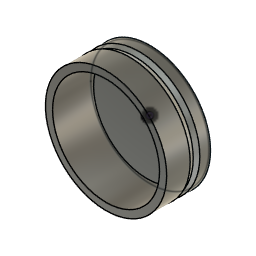
LW_AS_37_0150 (Autodesk Fusion 360 design; units mm, degrees)
Autodesk Fusion 360 part; units mm, degrees
sketch "Sketch1" plane through (0, 0, 0) normal (0, 0, 1) x (1, 0, 0)
  line L0 (0, 0) -> (17, 0)
  line L1 (17, 0) -> (17, -3)
  line L2 (17, -3) -> (17, -5.7)
  line L3 (17, -5.7) -> (17, -12.3)
  line L4 (17, -12.3) -> (15, -12.3)
  line L5 (15, -12.3) -> (15, -0.8)
  line L6 (17, -3) -> (17, -4.35) construction
  line L7 (17, -4.35) -> (16.5, -4.35) construction
  line L8 (17, -3) -> (16.5, -4.35)
  line L9 (16.5, -4.35) -> (17, -5.7)
  line L10 (0, 0) -> (0, -0.8)
  line L11 (0, -0.8) -> (15, -0.8)
  dimension "d1" = 17
  dimension "d2" = 3
  dimension "d4" = 2.7
  dimension "d5" = 6.6
  dimension "d6" = 2
  dimension "d8" = 1.35
  dimension "d9" = 0.5
  dimension "d10" = 15
  dimension "d12" = 17
  dimension "d19" = 0.8
  constraint coincident L0.start L10.start
  constraint horizontal L0
  constraint perpendicular L0 L1
  constraint parallel L1 L2
  constraint parallel L2 L3
  constraint perpendicular L3 L4
  constraint perpendicular L0 L5
  constraint coincident L2 L6.end
  constraint perpendicular L2 L7
  constraint perpendicular L0 L10
  constraint perpendicular L5 L11
  measures "d1" distance of L0.start L0.end
  measures "d2" distance of L0.end L1.end
  measures "d4" distance of L1.end L2.end
  measures "d5" distance of L2.end L3.end
  measures "d6" distance of L3.end L4.end
  measures "d8" distance of L1.end L6.end
  measures "d9" distance of L6.end L7.end
  measures "d10" distance of L5.end L10.end
  measures "d12" distance of L0.start L0.end
  measures "d19" distance of L0.start L10.end
revolve "Revolve1" add sketch "Sketch1" angle 360 about axis through (0, 0, 0) along (0, -1, 0) contours L0 L1 L3 L4 L5 L8 L9 L10 L11
sketch "Sketch2" plane through (0, 0, 0) normal (0, 1, 0) x (-1, 0, 0)
  circle A0 centre (0, 0) radius 17
  circle A1 centre (0, 0) radius 16.575
  circle A2 centre (0, 0) radius 0.75
  dimension "d14" = 34
  dimension "d15" = 33.15
  dimension "d16" = 1.5
  constraint coincident A0.centre A1.centre
  constraint concentric A1 A2
  measures "d14" diameter of A0
  measures "d15" diameter of A1
  measures "d16" diameter of A2
extrude "Extrude1" cut sketch "Sketch2" against normal blind 3 contours A2
equation "d15 = d14 - 0.85 mm"
